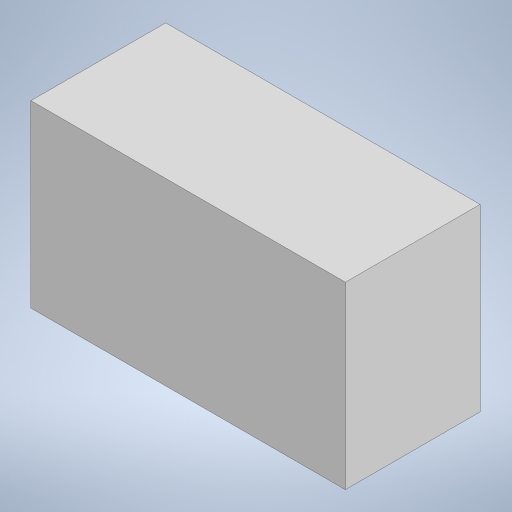
# Autodesk Inventor part: bearing_10
Saved by Autodesk Inventor 2024.3 (Build 283343000, 343)
## iProperties
Created: 2025-01-05
Part Number: bearing_10
Material: 一般
Document SubType Name: Modeling
Designer: 佐藤智貴
Density: 1 g/cm^3
Appearance: 既定
Author: 佐藤智貴
Autodesk Inventor part; units mm, degrees
ref_plane "YZ Plane" through (0, 0, 0) normal (1, 0, 0) x (0, 1, 0)
ref_plane "XZ Plane" through (0, 0, 0) normal (0, 1, 0) x (-1, 0, 0)
ref_plane "XY Plane" through (0, 0, 0) normal (0, 0, 1) x (1, 0, 0)
sketch "スケッチ1" plane through (0, 0, 0) normal (0, 0, 1) x (1, 0, 0)
  line L0 (0, 0) -> (350, 0)
  line L1 (350, 0) -> (350, 200)
  line L2 (350, 200) -> (0, 200)
  line L3 (0, 200) -> (0, 0)
  dimension "d0" = 350
  dimension "d1" = 200
  constraints: 8 end point, 2 parallel, 1 horizontal, 1 perpendicular
  measures "d0" distance of L1.end L2.end
  measures "d1" distance of L0.end L1.end
extrude "押し出し1" add sketch "スケッチ1" along normal blind 150
sketch "スケッチ2" plane through (0, 0, 0) normal (0, 0, -1) x (-1, 0, 0)
  circle A0 centre (-300, 50) radius 2.5
  circle A1 centre (-50, 50) radius 2.5
  line L0 (0, 0) -> (-350, 0) projected
  line L1 (-350, 0) -> (-350, 200) projected
  dimension "d4" = 50
  dimension "d5" = 50
  dimension "d6" = 250
  dimension "d7" = 50
  dimension "d8" = 5
  dimension "d9" = 5
  constraints: 2 centre point
  measures "d4" distance from line of L0 A0.centre
  measures "d5" distance from line of L0 A1.centre
  measures "d6" distance of A1.centre A0.centre
  measures "d7" distance from line of L1 A0.centre
  measures "d8" diameter of A0
  measures "d9" diameter of A1
extrude "押し出し2" add sketch "スケッチ2" along normal blind 1
equation "\"d5\" = d4"
equation "\"d9\" = d8"
